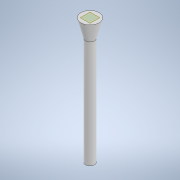
# Autodesk Inventor part: ramie
Saved by Autodesk Inventor 2021 (Build 250183000, 183)
## iProperties
Created: 2021-10-29
Part Number: ramie
Material: Generic
Document SubType Name: Modeling
Designer: nikod
Density: 1 g/cm^3
Appearance: Default
Mass: 13090 g
Surface Area: 5134.09 cm^2
Volume: 13090 cm^3
Author: nikod
Autodesk Inventor part; units mm, degrees
ref_plane "YZ Plane" through (0, 0, 0) normal (1, 0, 0) x (0, 1, 0)
ref_plane "XZ Plane" through (0, 0, 0) normal (0, 1, 0) x (-1, 0, 0)
ref_plane "XY Plane" through (0, 0, 0) normal (0, 0, 1) x (1, 0, 0)
sketch "Sketch1" plane through (0, 0, 0) normal (0, 1, 0) x (-1, 0, 0)
  circle A0 centre (0, 0) radius 50
  dimension "d0" = 100
  constraints: 1 centre point, 1 coincident
  measures "d0" diameter of A0
extrude "Extrusion1" add sketch "Sketch1" along normal blind 1200
ref_plane "Work Plane1" through (0, 1400, 0) normal (0, -1, 0) x (1, 0, 0)
sketch "Sketch2" plane through (0, 1400, 0) normal (0, -1, 0) x (1, 0, 0)
  circle A0 centre (0, 0) radius 100
  dimension "d4" = 200
  constraints: 1 centre point, 1 coincident
  measures "d4" diameter of A0
loft "Loft1" add profiles "Sketch2" section 1 edges at (50, 1200, 0)
body "Solid1"
